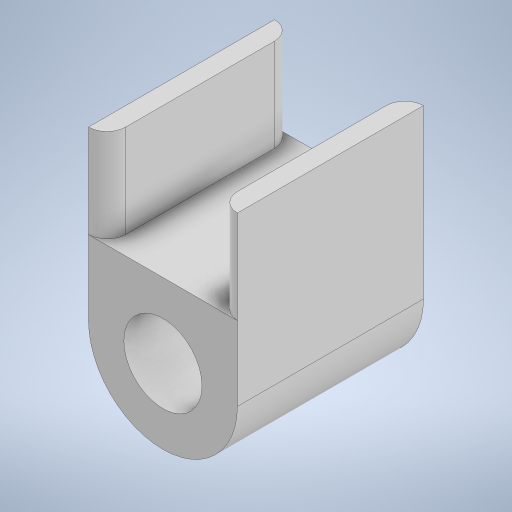
# Autodesk Inventor part: gomu_guide
Saved by Autodesk Inventor 2024 (Build 280153000, 153)
## iProperties
Created: 2024-07-18
Part Number: gomu_guide
Material: 一般
Document SubType Name: Modeling
Designer: Akio
Density: 1 g/cm^3
Appearance: 既定
Author: Akio
Autodesk Inventor part; units mm, degrees
ref_plane "YZ Plane" through (0, 0, 0) normal (1, 0, 0) x (0, 1, 0)
ref_plane "XZ Plane" through (0, 0, 0) normal (0, 1, 0) x (-1, 0, 0)
ref_plane "XY Plane" through (0, 0, 0) normal (0, 0, 1) x (1, 0, 0)
sketch "スケッチ1" plane through (0, 0, 0) normal (0, 1, 0) x (-1, 0, 0)
  line L0 (0, 0) -> (-4, 0)
  line L1 (-4, 0) -> (-4, -5)
  line L2 (-4, -5) -> (0, -5)
  line L3 (0, -5) -> (0, 0)
  dimension "d0" = 4
  dimension "d1" = 5
  constraints: 8 end point, 2 parallel, 1 horizontal, 1 perpendicular
  measures "d0" distance of L2.end L1.end
  measures "d1" distance of L1.end L0.end
extrude "押し出し1" add sketch "スケッチ1" along normal blind 6.5
sketch "スケッチ2" plane through (0, 0, 0) normal (0, 0, 1) x (1, 0, 0)
  line L0 (0, 0) -> (4, 0) projected
  line L1 (0, 0) -> (0, 6.5) projected
  point P0 (2, 2)
  dimension "d11" = 2
  dimension "d12" = 2
  measures "d11" distance from line of L0 point (2, 2)
  measures "d12" distance from line of L1 point (2, 2)
hole "穴1" at (2, 2, 0) direction (0, 0, -1) diameter 2.1 end through all
sketch "スケッチ3" plane through (0, 0, 0) normal (0, 0, 1) x (1, 0, 0)
  line L0 (0.5, 6.5) -> (3.5, 6.5)
  line L1 (3.5, 6.5) -> (3.5, 4)
  line L2 (3.5, 4) -> (0.5, 4)
  line L3 (0.5, 4) -> (0.5, 6.5)
  line L4 (0.5, 6.5) -> (3.5, 4) construction
  line L5 (3.5, 6.5) -> (0.5, 4) construction
  line L6 (0, 0) -> (0, 6.5) projected
  line L7 (0, 6.5) -> (4, 6.5) projected
  point P0 (2, 5.25)
  dimension "d13" = 3
  dimension "d14" = 2.5
  dimension "d15" = 2
  dimension "d16" = 0
  constraints: 12 end point, 2 midpoint, 2 parallel, 1 horizontal, 1 perpendicular
  measures "d13" distance of L1.end L2.end
  measures "d14" distance of L0.end L1.end
  measures "d15" distance from line of L6 point (2, 5.25)
  measures "d16" distance between parallel lines of L0 L7
extrude "押し出し2" cut sketch "スケッチ3" against normal through all
fillet "フィレット1" radius 2 2 edges at (4, 0, -2.5) (0, 0, -2.5)
fillet "フィレット2" radius 0.5 4 edges at (0.5, 5.25, 0) (3.5, 5.25, 0) (0.5, 5.25, -5) (3.5, 5.25, -5)
equation "\"d12\" = 0.5 * d0"
equation "\"d15\" = 0.5 * d0"
